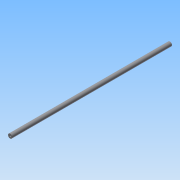
# Autodesk Inventor part: вал 8мм
Saved by Autodesk Inventor 2017 (Build 210142000, 142)
## iProperties
Part Number: вал 8мм
Material: Типовые
Document SubType Name: Modeling
Designer: Max
Mass: 16.5093 g
Surface Area: 84.7506 cm^2
Volume: 16.5093 cm^3
Density: 1 g/cm^3
Appearance: Сталь — полированная
Author: Max
Autodesk Inventor part; units mm, degrees
ref_plane "YZ Plane" through (0, 0, 0) normal (1, 0, 0) x (0, 1, 0)
ref_plane "XZ Plane" through (0, 0, 0) normal (0, 1, 0) x (-1, 0, 0)
ref_plane "XY Plane" through (0, 0, 0) normal (0, 0, 1) x (1, 0, 0)
sketch "Эскиз1" plane through (0, 0, 0) normal (0, 1, 0) x (-1, 0, 0)
  circle A0 centre (0, 0) radius 4
  dimension "d0" = 8
  constraints: 1 centre point, 1 coincident
  measures "d0" diameter of A0
extrude "Выдавливание1" add sketch "Эскиз1" along normal mid plane 329.9
sketch "Эскиз2" plane through (0, 164.95, 0) normal (0, 1, 0) x (1, 0, 0)
  circle A0 centre (0, 0) radius 1.5
  dimension "d3" = 3
  constraints: 1 centre point, 1 coincident
  measures "d3" diameter of A0
extrude "Выдавливание2" cut sketch "Эскиз2" against normal blind 5
mirror "Зеркальное отражение1" about plane through (0, 0, 0) normal (0, 1, 0) of "Выдавливание2"
fillet "Сопряжение1" radius 0.5 2 edges at (4, -164.95, 0) (4, 164.95, 0)
